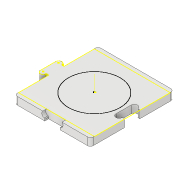
# Autodesk Inventor part: 10_Base_puzzle_sideplate_v3
Saved by Autodesk Inventor 2022 (Build 260153000, 153)
## iProperties
Created: 2017-06-20
Part Number: 10_Base_puzzle_sideplate_v3
Material: Generisch
Document SubType Name: Modeling
Designer: diederichbenedict
Density: 1 g/cm^3
Appearance: Weiß
Mass: 7.87446 g
Surface Area: 71.4468 cm^2
Volume: 7.87446 cm^3
d_part: 50,000 mm
d_o: 40,000 mm
d_i: 40,000 mm
Author: diederichbenedict
Autodesk Inventor part; units mm, degrees
ref_plane "YZ Plane" through (0, 0, 0) normal (1, 0, 0) x (0, 1, 0)
ref_plane "XZ Plane" through (0, 0, 0) normal (0, 1, 0) x (-1, 0, 0)
ref_plane "XY Plane" through (0, 0, 0) normal (0, 0, 1) x (1, 0, 0)
sketch "Skizze1" plane through (0, 0, 0) normal (0, 0, 1) x (1, 0, 0)
  line L0 (-17.4, -0.2) -> (-25.4, -0.2)
  line L1 (-25.4, -0.2) -> (-25.4, -23.2)
  line L2 (-23.4, -25.2) -> (-0.4, -25.2)
  line L3 (-0.4, -25.2) -> (-0.4, -17.2)
  line L4 (-17.4, -0.2) -> (-17.4, -15.2)
  line L5 (-15.4, -17.2) -> (-0.4, -17.2)
  arc A0 (-25.4, -23.2) -> (-23.4, -25.2) centre (-23.4, -23.2) ccw
  circle A1 centre (-20.4, -20.2) radius 2.425
  circle A2 centre (-21.2, -14.7) radius 2.65
  circle A3 centre (-14.9, -21) radius 2.65
  arc A4 (-17.4, -15.2) -> (-15.4, -17.2) centre (-15.4, -15.2) ccw
  circle A5 centre (-20.4, -20.2) radius 2.425
  circle A6 centre (-14.9, -21) radius 2.65
  circle A7 centre (-21.2, -14.7) radius 2.65
  line L6 (-17.4, -0.2) -> (-0.4, -0.2)
  line L7 (-0.4, -0.2) -> (-0.4, -17.2)
  line L8 (-25.4, -23.2) -> (-25.4, -25.2)
  line L9 (-25.4, -25.2) -> (-23.4, -25.2)
  point P0 (-17.4, -17.2)
  dimension "d278" = 25
  dimension "d279" = 25
  dimension "d2" = 8
  dimension "d281" = 8
  dimension "d282" = 2
  dimension "d283" = 4.85
  dimension "d284" = 20
  dimension "d4" = 20
  dimension "d286" = 5.3
  dimension "d_hole" = 5.3
  dimension "d290" = 20.8
  dimension "d" = 20.8
  dimension "d292" = 2
  dimension "d313" = 6.3
  dimension "d314" = 6.3
  dimension "d330" = 0
  dimension "d331" = 0
  dimension "d332" = 0
  constraints: 20 end point, 8 centre point, 5 tangent, 4 point on circle, 4 point on line, 3 horizontal, 2 coincident, 2 parallel, 1 collinear, 1 perpendicular, 1 vertical
  measures "d278" distance of L2.end L8.end
  measures "d279" distance of L8.end L0.end
  measures "d2" distance between parallel lines of L4 L1
  measures "d281" distance between parallel lines of L2 L5
  measures "d282" radius of A0
  measures "d283" diameter of A1
  measures "d284" distance from line of L0 A1.centre
  measures "d4" distance from line of L3 A1.centre
  measures "d286" diameter of A2
  measures "d_hole" diameter of A3
  measures "d290" distance from line of L0 A3.centre
  measures "d" distance from line of L3 A2.centre
  measures "d292" radius of A4
  measures "d313" horizontal distance of A2.centre A3.centre
  measures "d314" horizontal distance of A2.centre A3.centre
  measures "d330" radial gap between concentric circles of A1 A5
  measures "d331" radial gap between concentric circles of A3 A6
  measures "d332" radial gap between concentric circles of A2 A7
extrude "Extrusion1" add sketch "Skizze1" along normal blind 5 contours L4 A4 L5 L3 L2 A0 L1 L0 | L6 L7 L5 A4 L4 | A0 L9 L8 | A1 | A2 | A3
mirror "Mirror6" about plane through (-17.4, -0.2, 0) normal (0, 1, 0) of "Extrusion1"
mirror "Mirror7" about plane through (-0.4, -25.2, 0) normal (1, 0, 0) of "Extrusion1", "Mirror6"
sketch "Sketch26" plane through (0, 0, 5) normal (0, 0, 1) x (1, 0, 0)
  line L0 (24.6, 24.8) -> (-25.4, 24.8) projected
  line L1 (-25.4, -25.2) -> (-25.4, 24.8) projected
  line L2 (-25.4, -25.2) -> (24.6, -25.2) projected
  line L3 (24.6, 24.8) -> (24.6, -25.2) projected
  line L4 (-25.4, -23.2) -> (-25.4, 22.8) projected
  line L5 (-28.9, -7.2) -> (-28.9, -7.2)
  line L6 (-30.9, -5.2) -> (-30.9, 4.8)
  line L7 (-28.9, 6.8) -> (-28.9, 6.8)
  line L8 (-25.4, 6.8) -> (-25.4, -7.2)
  line L9 (-26.9, -5.2) -> (-26.9, 4.8)
  line L10 (-26.4505, 4.8) -> (-25.4, 4.8)
  line L11 (-25.4, 4.8) -> (-25.4, -5.2)
  line L12 (-25.4, -5.2) -> (-26.4505, -5.2)
  line L13 (-26.9, -5.2) -> (-25.4, 4.8) construction
  line L14 (-26.9, 4.8) -> (-25.4, -5.2) construction
  line L15 (-26.9, -5.2) -> (-26.9, -5.2)
  line L16 (-26.9, 4.8) -> (-26.9, 4.8)
  arc A0 (-30.9, -5.2) -> (-28.9, -7.2) centre (-28.9, -5.2) ccw
  arc A1 (-28.9, -7.2) -> (-26.9404, -5.6) centre (-28.9, -5.2) ccw
  arc A2 (-28.9, 6.8) -> (-30.9, 4.8) centre (-28.9, 4.8) ccw
  arc A3 (-26.9404, 5.2) -> (-28.9, 6.8) centre (-28.9, 4.8) ccw
  arc A4 (-26.4505, -5.2) -> (-26.9404, -5.6) centre (-26.4505, -5.7) ccw
  arc A5 (-26.9404, 5.2) -> (-26.4505, 4.8) centre (-26.4505, 5.3) ccw
  point P0 (0, 0)
  point P1 (-26.15, -0.2)
  point P2 (-25.4, -0.2)
  dimension "d293" = 5.5
  dimension "d294" = 14
  dimension "d295" = 18
  dimension "d296" = 10
  dimension "d297" = 1.5
  dimension "d300" = 2
  dimension "d301" = 0.5
  constraints: 24 end point, 14 point on circle, 12 tangent, 6 centre point, 4 equal radius, 4 midpoint, 4 parallel, 3 perpendicular, 3 point on line, 1 horizontal, 1 vertical
  measures "d293" distance between parallel lines of L1 L6
  measures "d294" distance between parallel lines of L5 L7
  measures "d295" distance between parallel lines of L7 L0
  measures "d296" distance of L9.start L9.end
  measures "d297" distance of L9.end L10.end
  measures "d300" radius of A0
  measures "d301" radius of A4
extrude "Extrusion13" add sketch "Sketch26" against normal up to surface (5 mm away) contours L1 L12 A4 A1 A0 L6 A2 A3 A5 L10
sketch "Sketch27" plane through (0, 0, 5) normal (0, 0, 1) x (1, 0, 0)
  line L0 (24.6, 24.8) -> (-25.4, 24.8) projected
  line L1 (-25.4, -25.2) -> (-25.4, -5.2) projected
  line L2 (-26.4505, 4.8) -> (-25.4, 4.8) projected
  arc A0 (-26.9404, 5.2) -> (-26.4505, 4.8) centre (-26.4505, 5.3) ccw projected
  arc A1 (-26.9404, 5.2) -> (-30.9, 4.8) centre (-28.9, 4.8) ccw projected
  line L3 (-30.9, -5.2) -> (-30.9, 4.8) projected
  arc A2 (-30.9, -5.2) -> (-26.9404, -5.6) centre (-28.9, -5.2) ccw projected
  arc A3 (-26.4505, -5.2) -> (-26.9404, -5.6) centre (-26.4505, -5.7) ccw projected
  line L4 (-25.4, -5.2) -> (-26.4505, -5.2) projected
  line L5 (-25.4, 4.8) -> (-25.4, 24.8) projected
  line L6 (-25.4, -25.2) -> (24.6, -25.2) projected
  line L7 (24.6, 24.8) -> (24.6, -25.2) projected
  circle A4 centre (-0.4, -0.2) radius 17
  point P0 (0, 0)
  constraints: 1 centre point
sketch "Sketch28" plane through (0, 0, 5) normal (0, 0, 1) x (1, 0, 0)
  line L0 (24.6, 24.8) -> (-25.4, 24.8) projected
  line L1 (-25.4, -25.2) -> (-25.4, -5.2) projected
  line L2 (-26.4505, 4.8) -> (-25.4, 4.8) projected
  arc A0 (-26.9404, 5.2) -> (-26.4505, 4.8) centre (-26.4505, 5.3) ccw projected
  arc A1 (-26.9404, 5.2) -> (-30.9, 4.8) centre (-28.9, 4.8) ccw projected
  line L3 (-30.9, -5.2) -> (-30.9, 4.8) projected
  arc A2 (-30.9, -5.2) -> (-26.9404, -5.6) centre (-28.9, -5.2) ccw projected
  arc A3 (-26.4505, -5.2) -> (-26.9404, -5.6) centre (-26.4505, -5.7) ccw projected
  line L4 (-25.4, -5.2) -> (-26.4505, -5.2) projected
  line L5 (-25.4, 4.8) -> (-25.4, 24.8) projected
  line L6 (-25.4, -25.2) -> (24.6, -25.2) projected
  line L7 (24.6, 24.8) -> (24.6, -25.2) projected
  line L8 (-25.4, 22.8) -> (-25.4, 4.8) projected
  line L9 (-25.4, -5.2) -> (-25.4, 4.8)
  line L10 (-30.9, -5.2) -> (-30.9, 4.8)
  arc A4 (-30.9, -5.2) -> (-26.9687, -5.7197) centre (-28.9, -5.2) ccw
  arc A5 (-26.9404, 5.2) -> (-30.9, 4.8) centre (-28.9, 4.8) ccw
  line L11 (-25.4, -5.2) -> (-26.2523, -5.2)
  line L12 (-25.4, 4.8) -> (-26.4505, 4.8)
  arc A6 (-26.2523, -5.2) -> (-25.9588, -5.6095) centre (-25.7545, -5.1531) ccw
  arc A7 (-26.9404, 5.2) -> (-26.4505, 4.8) centre (-26.4505, 5.3) ccw
  arc A8 (-26.9404, 5.2) -> (-26.4505, 4.8) centre (-26.4505, 5.3) ccw projected
  line L13 (-26.9404, 5.2) -> (-26.9404, 5.2)
  line L14 (-26.9687, -5.7197) -> (-25.9588, -5.6095)
  line L15 (24.527, -5.0054) -> (24.527, 4.8151)
  line L16 (19.0089, -5.0023) -> (19.0089, 4.8)
  arc A9 (19.0089, -5.0023) -> (22.9683, -5.5256) centre (20.997, -5.2) ccw
  arc A10 (22.9981, 5.203) -> (19.0089, 4.8) centre (21.0238, 4.8) ccw
  line L17 (24.527, -5.0054) -> (23.4703, -5.0054)
  line L18 (24.527, 4.8151) -> (23.4731, 4.8151)
  arc A11 (23.4703, -5.0054) -> (22.9989, -5.4045) centre (23.4777, -5.4921) ccw
  arc A12 (22.9977, 5.2047) -> (23.4731, 4.8151) centre (23.4731, 5.2998) ccw
  line L19 (22.9977, 5.2047) -> (22.9981, 5.203)
  line L20 (22.9683, -5.5256) -> (22.9989, -5.4045)
  line L21 (18.9339, 4.8) -> (18.9339, -4.9986)
  arc A13 (18.9339, -4.9986) -> (23.0417, -5.541) centre (20.997, -5.2) ccw
  line L22 (23.0417, -5.541) -> (23.0722, -5.4203)
  arc A14 (23.4709, -5.0804) -> (23.0722, -5.4203) centre (23.4777, -5.4921) ccw
  line L23 (23.4709, -5.0804) -> (24.602, -5.0804)
  line L24 (24.602, -5.0804) -> (24.602, 4.8901)
  line L25 (24.602, 4.8901) -> (23.4731, 4.8901)
  arc A15 (23.0716, 5.2179) -> (23.4731, 4.8901) centre (23.4731, 5.2998) ccw
  arc A16 (23.0716, 5.2179) -> (18.9339, 4.8) centre (21.0238, 4.8) ccw
  point P0 (0, 0)
  dimension "d307" = 0.075
  dimension "d315" = 0.1946
  dimension "d316" = 0
  dimension "d317" = 0
  dimension "d318" = 0.0901
  constraints: 34 end point, 28 point on circle, 12 centre point, 5 tangent, 4 parallel, 4 vertical, 1 equal radius, 1 point on line, 8 other
  measures "d307" radial gap between concentric circles of A10 A16
  measures "d315" distance between parallel lines of L11 L17
  measures "d316" vertical distance of A9.centre A2.centre
  measures "d317" vertical distance of A10.centre A5.centre
  measures "d318" distance between parallel lines of L2 L25
extrude "Extrusion14" cut sketch "Sketch28" against normal blind 10 contours L7 L23 A14 L22 A13 L21 A16 A15 L25 | L17 A11 L20 A9 L16 A10 A12 L18 L15
sketch "Sketch30" plane through (0, 0, 5) normal (0, 0, 1) x (1, 0, 0)
  line L0 (24.6, 24.8) -> (-25.4, 24.8) construction
  line L1 (-25.4, -25.2) -> (-25.4, -5.2) construction
  line L2 (-26.4505, 4.8) -> (-25.4, 4.8) construction
  arc A0 (-26.9404, 5.2) -> (-26.4505, 4.8) centre (-26.4505, 5.3) ccw construction
  arc A1 (-26.9404, 5.2) -> (-30.9, 4.8) centre (-28.9, 4.8) ccw construction
  line L3 (-30.9, -5.2) -> (-30.9, 4.8) construction
  arc A2 (-30.9, -5.2) -> (-26.9404, -5.6) centre (-28.9, -5.2) ccw construction
  arc A3 (-26.4505, -5.2) -> (-26.9404, -5.6) centre (-26.4505, -5.7) ccw construction
  line L4 (-25.4, -5.2) -> (-26.4505, -5.2) construction
  line L5 (-25.4, 4.8) -> (-25.4, 24.8) construction
  line L6 (-25.4, -25.2) -> (24.6, -25.2) construction
  line L7 (24.6, 24.8) -> (24.6, 4.8901) construction
  line L8 (24.6, -5.0804) -> (23.4709, -5.0804) construction
  arc A4 (23.4709, -5.0804) -> (23.0722, -5.4203) centre (23.4777, -5.4921) ccw construction
  line L9 (23.0722, -5.4203) -> (23.0417, -5.541) construction
  arc A5 (18.9339, -4.9986) -> (23.0417, -5.541) centre (20.997, -5.2) ccw construction
  line L10 (18.9339, -4.9986) -> (18.9339, 4.8) construction
  arc A6 (23.0716, 5.2179) -> (18.9339, 4.8) centre (21.0238, 4.8) ccw construction
  arc A7 (23.0716, 5.2179) -> (23.4731, 4.8901) centre (23.4731, 5.2998) ccw construction
  line L11 (23.4731, 4.8901) -> (24.6, 4.8901) construction
  line L12 (24.6, -5.0804) -> (24.6, -25.2) construction
  line L13 (-28.9, -7.2) -> (-28.9, -7.2)
  line L14 (-30.9, -5.2) -> (-30.9, 4.8)
  line L15 (-28.9, 6.8) -> (-28.9, 6.8)
  line L16 (-26.9, -5.2) -> (-26.9, 4.8)
  line L17 (-26.4505, 4.8) -> (-25.4, 4.8)
  line L18 (-25.4, 4.8) -> (-25.4, -5.2)
  line L19 (-25.4, -5.2) -> (-26.4505, -5.2)
  line L20 (-26.9, -5.2) -> (-25.4, 4.8) construction
  line L21 (-26.9, 4.8) -> (-25.4, -5.2) construction
  line L22 (-26.9, -5.2) -> (-26.9, -5.2)
  line L23 (-26.9, 4.8) -> (-26.9, 4.8)
  arc A8 (-30.9, -5.2) -> (-28.9, -7.2) centre (-28.9, -5.2) ccw
  arc A9 (-28.9, -7.2) -> (-26.9404, -5.6) centre (-28.9, -5.2) ccw
  arc A10 (-28.9, 6.8) -> (-30.9, 4.8) centre (-28.9, 4.8) ccw
  arc A11 (-26.9404, 5.2) -> (-28.9, 6.8) centre (-28.9, 4.8) ccw
  arc A12 (-26.4505, -5.2) -> (-26.9404, -5.6) centre (-26.4505, -5.7) ccw
  arc A13 (-26.9404, 5.2) -> (-26.4505, 4.8) centre (-26.4505, 5.3) ccw
  arc A14 (-28.9, 6.875) -> (-30.975, 4.8) centre (-28.9, 4.8) ccw
  line L24 (-30.975, 4.8) -> (-30.975, -5.2)
  arc A15 (-30.975, -5.2) -> (-29.5327, -7.1762) centre (-28.9, -5.2) ccw
  arc A16 (-29.5327, -7.1762) -> (-26.8669, -5.615) centre (-28.9, -5.2) ccw
  arc A17 (-26.4505, -5.275) -> (-26.8669, -5.615) centre (-26.4505, -5.7) ccw
  line L25 (-26.4505, -5.275) -> (-25.325, -5.275)
  line L26 (-25.325, -5.275) -> (-25.325, 4.875)
  line L27 (-25.325, 4.875) -> (-26.4505, 4.875)
  arc A18 (-26.8669, 5.215) -> (-26.4505, 4.875) centre (-26.4505, 5.3) ccw
  arc A19 (-26.8669, 5.215) -> (-28.9, 6.875) centre (-28.9, 4.8) ccw
  arc A20 (-28.9, 6.8) -> (-30.9, 4.8) centre (-28.9, 4.8) ccw
  line L28 (-30.9, 4.8) -> (-30.9, -5.2)
  arc A21 (-30.9, -5.2) -> (-29.5098, -7.1048) centre (-28.9, -5.2) ccw
  arc A22 (-29.5098, -7.1048) -> (-26.9404, -5.6) centre (-28.9, -5.2) ccw
  arc A23 (-26.4505, -5.2) -> (-26.9404, -5.6) centre (-26.4505, -5.7) ccw
  line L29 (-26.4505, -5.2) -> (-25.4, -5.2)
  line L30 (-25.4, 4.8) -> (-26.4505, 4.8)
  arc A24 (-26.9404, 5.2) -> (-26.4505, 4.8) centre (-26.4505, 5.3) ccw
  arc A25 (-26.9404, 5.2) -> (-28.9, 6.8) centre (-28.9, 4.8) ccw
  line L31 (-25.4, 4.8) -> (-25.4, -5.2)
  line L32 (-26.4505, 4.8) -> (-25.4, 4.8) projected
  line L33 (-25.4, 4.8) -> (-25.4, 4.8)
  line L34 (-25.4, -5.2) -> (-26.4505, -5.2) projected
  line L35 (-25.4, -5.2) -> (-25.4, -5.2)
  arc A26 (22.9977, 5.2047) -> (23.4731, 4.8151) centre (23.4731, 5.2998) ccw
  line L36 (24.527, -5.0054) -> (24.527, 4.8151)
  line L37 (19.0089, -5.0023) -> (19.0089, 4.8)
  line L38 (24.527, -5.0054) -> (23.4703, -5.0054)
  arc A27 (23.4703, -5.0054) -> (22.9989, -5.4045) centre (23.4777, -5.4921) ccw
  line L39 (22.9683, -5.5256) -> (22.9989, -5.4045)
  arc A28 (19.0089, -5.0023) -> (22.9683, -5.5256) centre (20.997, -5.2) ccw
  line L40 (24.527, 4.8151) -> (23.4731, 4.8151)
  line L41 (22.9977, 5.2047) -> (22.9981, 5.203)
  arc A29 (22.9981, 5.203) -> (19.0089, 4.8) centre (21.0238, 4.8) ccw
  line L42 (18.8989, 4.8) -> (18.8989, -4.9969)
  arc A30 (18.8989, -4.9969) -> (23.076, -5.5482) centre (20.997, -5.2) ccw
  line L43 (23.076, -5.5482) -> (23.1065, -5.4276)
  arc A31 (23.4712, -5.1154) -> (23.1065, -5.4276) centre (23.4777, -5.4921) ccw
  line L44 (23.4712, -5.1154) -> (24.637, -5.1154)
  line L45 (24.637, -5.1154) -> (24.637, 4.9251)
  line L46 (24.637, 4.9251) -> (23.4731, 4.9251)
  arc A32 (23.1059, 5.2249) -> (23.4731, 4.9251) centre (23.4731, 5.2998) ccw
  arc A33 (23.1059, 5.2249) -> (18.8989, 4.8) centre (21.0238, 4.8) ccw
  line L47 (24.637, 4.9251) -> (24.637, -5.1154)
  line L48 (24.637, -5.1154) -> (23.4712, -5.1154)
  arc A34 (23.4712, -5.1154) -> (23.1065, -5.4276) centre (23.4777, -5.4921) ccw
  line L49 (23.1065, -5.4276) -> (23.076, -5.5482)
  arc A35 (18.8989, -4.9969) -> (23.076, -5.5482) centre (20.997, -5.2) ccw
  line L50 (18.8989, -4.9969) -> (18.8989, 4.8)
  arc A36 (23.1059, 5.2249) -> (18.8989, 4.8) centre (21.0238, 4.8) ccw
  arc A37 (23.1059, 5.2249) -> (23.4731, 4.9251) centre (23.4731, 5.2998) ccw
  line L51 (23.4731, 4.9251) -> (24.637, 4.9251)
  point P0 (-26.15, -0.2)
  point P1 (-25.4, -0.2)
  dimension "d334" = 14
  dimension "d336" = 10
  dimension "d337" = 1.5
  dimension "d338" = 2
  dimension "d339" = 0.5
  dimension "d340" = 0.075
  dimension "d341" = 0.075
  dimension "d342" = 0.075
  dimension "d343" = 0.075
  dimension "d346" = 0.11
  dimension "d347" = 0
  constraints: 74 end point, 62 point on circle, 30 centre point, 13 tangent, 9 vertical, 8 parallel, 4 equal radius, 3 horizontal, 3 midpoint, 3 perpendicular, 2 collinear, 2 point on line, 38 other
  measures "d334" distance between parallel lines of L13 L15
  measures "d336" distance of L16.start L16.end
  measures "d337" distance of L16.end L17.end
  measures "d338" radius of A8
  measures "d339" radius of A12
  measures "d340" radial gap between concentric circles of A11 A19
  measures "d341" radial gap between concentric circles of A19 A25
  measures "d342" distance between parallel lines of L24 L28
  measures "d343" radial gap between concentric circles of A16 A22
  measures "d346" radial gap between concentric circles of A29 A33
  measures "d347" distance between parallel lines of L45 L47
extrude "Extrusion15" cut sketch "Sketch30" against normal blind 10 contours A26 L40 L36 L38 A27 L39 A28 L37 A29 | A33 A32 L46 L45 L44 A31 L43 A30 L42
sketch "Skizze32" plane through (-23.4, 24.8, 5) normal (0, 1, 0) x (1, 0, 0)
  line L0 (-2, 5) -> (48, 5) projected
  line L1 (48, 0) -> (-2, 0) projected
  circle A0 centre (2, 29.8) radius 2.5 projected
  circle A1 centre (23.4, 51) radius 2.5 projected
  line L2 (27.8804, 6.1291) -> (27.8804, 5) projected
  line L3 (27.8804, 5) -> (46, 5) projected
  arc A2 (46, 5) -> (48, 7) centre (46, 7) ccw projected
  line L4 (48, 24.9099) -> (48, 7) projected
  line L5 (48, 24.9099) -> (46.8731, 24.9099) projected
  arc A3 (46.8731, 24.9099) -> (46.4716, 24.5821) centre (46.8731, 24.5002) ccw projected
  arc A4 (42.3339, 25) -> (46.4716, 24.5821) centre (44.4238, 25) ccw projected
  line L6 (42.3339, 25) -> (42.3339, 34.7986) projected
  arc A5 (46.4417, 35.341) -> (42.3339, 34.7986) centre (44.397, 35) ccw projected
  line L7 (46.4417, 35.341) -> (46.4722, 35.2203) projected
  arc A6 (46.4722, 35.2203) -> (46.8709, 34.8804) centre (46.8777, 35.2921) ccw projected
  line L8 (46.8709, 34.8804) -> (48, 34.8804) projected
  line L9 (48, 53) -> (48, 34.8804) projected
  arc A7 (48, 53) -> (46, 55) centre (46, 53) ccw projected
  line L10 (46, 55) -> (28, 55) projected
  line L11 (28, 55) -> (28, 56.0505) projected
  arc A8 (28.4, 56.5404) -> (28, 56.0505) centre (28.5, 56.0505) ccw projected
  arc A9 (28.4, 56.5404) -> (28, 60.5) centre (28, 58.5) ccw projected
  line L12 (28, 60.5) -> (18, 60.5) projected
  arc A10 (18, 60.5) -> (17.6, 56.5404) centre (18, 58.5) ccw projected
  arc A11 (18, 56.0505) -> (17.6, 56.5404) centre (17.5, 56.0505) ccw projected
  line L13 (18, 56.0505) -> (18, 55) projected
  line L14 (18, 55) -> (0, 55) projected
  arc A12 (0, 55) -> (-2, 53) centre (0, 53) ccw projected
  line L15 (-2, 35) -> (-2, 53) projected
  line L16 (-2, 35) -> (-3.0505, 35) projected
  arc A13 (-3.5404, 35.4) -> (-3.0505, 35) centre (-3.0505, 35.5) ccw projected
  arc A14 (-3.5404, 35.4) -> (-7.5, 35) centre (-5.5, 35) ccw projected
  line L17 (-7.5, 35) -> (-7.5, 25) projected
  arc A15 (-7.5, 25) -> (-3.5404, 24.6) centre (-5.5, 25) ccw projected
  arc A16 (-3.0505, 25) -> (-3.5404, 24.6) centre (-3.0505, 24.5) ccw projected
  line L18 (-3.0505, 25) -> (-2, 25) projected
  line L19 (-2, 7) -> (-2, 25) projected
  arc A17 (-2, 7) -> (0, 5) centre (0, 7) ccw projected
  line L20 (0, 5) -> (17.9099, 5) projected
  line L21 (17.9099, 5) -> (17.9099, 6.1269) projected
  arc A18 (17.9099, 6.1269) -> (17.5821, 6.5284) centre (17.5002, 6.1269) ccw projected
  arc A19 (18, 10.6661) -> (17.5821, 6.5284) centre (18, 8.5762) ccw projected
  line L22 (18, 10.6661) -> (27.7986, 10.6661) projected
  arc A20 (28.341, 6.5583) -> (27.7986, 10.6661) centre (28, 8.603) ccw projected
  line L23 (28.341, 6.5583) -> (28.2203, 6.5278) projected
  arc A21 (28.2203, 6.5278) -> (27.8804, 6.1291) centre (28.2921, 6.1223) ccw projected
  line L24 (8, 13) -> (38, 13) projected
  arc A22 (6, 15) -> (8, 13) centre (8, 15) ccw projected
  line L25 (6, 15) -> (6, 45) projected
  arc A23 (8, 47) -> (6, 45) centre (8, 45) ccw projected
  line L26 (8, 47) -> (38, 47) projected
  arc A24 (40, 45) -> (38, 47) centre (38, 45) ccw projected
  line L27 (40, 45) -> (40, 15) projected
  arc A25 (38, 13) -> (40, 15) centre (38, 15) ccw projected
  circle A26 centre (43, 10) radius 2.425 projected
  circle A27 centre (37.5, 9.2) radius 2.65 projected
  circle A28 centre (43.8, 15.5) radius 2.65 projected
  circle A29 centre (43, 50) radius 2.425 projected
  circle A30 centre (37.5, 50.8) radius 2.65 projected
  circle A31 centre (43.8, 44.5) radius 2.65 projected
  circle A32 centre (3, 10) radius 2.425 projected
  circle A33 centre (8.5, 9.2) radius 2.65 projected
  circle A34 centre (2.2, 15.5) radius 2.65 projected
  circle A35 centre (2.2, 44.5) radius 2.65 projected
  circle A36 centre (8.5, 50.8) radius 2.65 projected
  circle A37 centre (3, 50) radius 2.425 projected
  line L28 (-2, 5) -> (-2, 0) projected
  line L29 (48, 5) -> (48, 0) projected
  line L30 (-2, 0) -> (48, 0)
  line L31 (48, 0) -> (48, 5)
  line L32 (48, 5) -> (-2, 5)
  line L33 (-2, 5) -> (-2, 0)
  line L34 (-2, 5) -> (-2, 0) projected
  line L35 (48, 5) -> (48, 0) projected
  arc A38 (17.9849, 6.1269) -> (17.5971, 6.6019) centre (17.5002, 6.1269) ccw
  line L36 (17.9849, 6.1269) -> (17.9849, 4.925)
  line L37 (17.9849, 4.925) -> (0, 4.925)
  arc A39 (-2.075, 7) -> (0, 4.925) centre (0, 7) ccw
  line L38 (-2.075, 7) -> (-2.075, 24.925)
  line L39 (-2.075, 24.925) -> (-3.0505, 24.925)
  arc A40 (-3.0505, 24.925) -> (-3.4669, 24.585) centre (-3.0505, 24.5) ccw
  arc A41 (-7.575, 25) -> (-3.4669, 24.585) centre (-5.5, 25) ccw
  line L40 (-7.575, 25) -> (-7.575, 35)
  arc A42 (-3.4669, 35.415) -> (-7.575, 35) centre (-5.5, 35) ccw
  arc A43 (-3.4669, 35.415) -> (-3.0505, 35.075) centre (-3.0505, 35.5) ccw
  line L41 (-3.0505, 35.075) -> (-2.075, 35.075)
  line L42 (-2.075, 35.075) -> (-2.075, 53)
  arc A44 (0, 55.075) -> (-2.075, 53) centre (0, 53) ccw
  line L43 (0, 55.075) -> (17.925, 55.075)
  line L44 (17.925, 55.075) -> (17.925, 56.0505)
  arc A45 (17.925, 56.0505) -> (17.585, 56.4669) centre (17.5, 56.0505) ccw
  arc A46 (18, 60.575) -> (17.585, 56.4669) centre (18, 58.5) ccw
  line L45 (18, 60.575) -> (28, 60.575)
  arc A47 (28.415, 56.4669) -> (28, 60.575) centre (28, 58.5) ccw
  arc A48 (28.415, 56.4669) -> (28.075, 56.0505) centre (28.5, 56.0505) ccw
  line L46 (28.075, 56.0505) -> (28.075, 55.075)
  line L47 (28.075, 55.075) -> (46, 55.075)
  arc A49 (48.075, 53) -> (46, 55.075) centre (46, 53) ccw
  line L48 (48.075, 53) -> (48.075, 34.8054)
  line L49 (48.075, 34.8054) -> (46.8703, 34.8054)
  arc A50 (46.3989, 35.2045) -> (46.8703, 34.8054) centre (46.8777, 35.2921) ccw
  line L50 (46.3989, 35.2045) -> (46.3683, 35.3256)
  arc A51 (46.3683, 35.3256) -> (42.4089, 34.8023) centre (44.397, 35) ccw
  line L51 (42.4089, 34.8023) -> (42.4089, 25)
  arc A52 (42.4089, 25) -> (46.3981, 24.5971) centre (44.4238, 25) ccw
  arc A53 (46.8731, 24.9849) -> (46.3981, 24.5971) centre (46.8731, 24.5002) ccw
  line L52 (46.8731, 24.9849) -> (48.075, 24.9849)
  line L53 (48.075, 24.9849) -> (48.075, 7)
  arc A54 (46, 4.925) -> (48.075, 7) centre (46, 7) ccw
  line L54 (46, 4.925) -> (27.8054, 4.925)
  line L55 (27.8054, 4.925) -> (27.8054, 6.1297)
  arc A55 (28.2045, 6.6011) -> (27.8054, 6.1297) centre (28.2921, 6.1223) ccw
  line L56 (28.2045, 6.6011) -> (28.3256, 6.6317)
  arc A56 (28.3256, 6.6317) -> (27.8023, 10.5911) centre (28, 8.603) ccw
  line L57 (27.8023, 10.5911) -> (18, 10.5911)
  arc A57 (18, 10.5911) -> (17.5971, 6.6019) centre (18, 8.5762) ccw
  point P0 (23.4, 5)
  point P1 (27.8054, 5)
  point P2 (17.9849, 5)
  point P3 (-2, 0)
  point P4 (48, 5)
  dimension "d359" = 0.075
  constraints: 52 end point, 40 point on circle, 20 centre point, 2 parallel, 1 horizontal, 1 perpendicular, 41 other
  measures "d359" radial gap between concentric circles of A19 A57
extrude "Extrusion17" add sketch "Skizze32" along normal blind 2.5 contours L0 L36 L37 A39 | A39 L37 L36 L0 L55 L54 A54 L29 L1 L28 | L36 A38 A57 L57 A56 L56 A55 L55 L0 | L0 A54 L54 L55
sketch "Skizze33" plane through (-23.4, -25.2, 0) normal (0, -1, 0) x (1, 0, 0)
  arc A0 (28.4, 1.5404) -> (28, 5.5) centre (28, 3.5) ccw projected
  line L0 (-2, 0) -> (48, 0) projected
  line L1 (-2, 5) -> (48, 5) projected
  line L2 (17.9849, 0) -> (27.8054, 0) projected
  line L3 (46, 0) -> (48, 0) projected
  line L4 (48, 0) -> (48, 5) projected
  line L5 (48, 5) -> (46, 5) projected
  line L6 (46, 0) -> (46, 5) projected
  line L7 (0, 0) -> (-2, 0) projected
  line L8 (0, 0) -> (0, 5) projected
  line L9 (-2, 5) -> (0, 5) projected
  line L10 (-2, 0) -> (-2, 5) projected
  circle A1 centre (2.2, -32.9227) radius 1.5 projected
  line L11 (38, -42) -> (8, -42) projected
  arc A2 (38, -42) -> (40, -40) centre (38, -40) ccw projected
  line L12 (40, -40) -> (40, -10) projected
  arc A3 (40, -10) -> (38, -8) centre (38, -10) ccw projected
  line L13 (23.4, -8) -> (38, -8) projected
  circle A4 centre (23.4, -4) radius 4 projected
  line L14 (8, -8) -> (23.4, -8) projected
  arc A5 (8, -8) -> (6, -10) centre (8, -10) ccw projected
  line L15 (6, -10) -> (6, -25.2) projected
  circle A6 centre (2, -25.2) radius 4 projected
  line L16 (6, -25.2) -> (6, -40) projected
  arc A7 (6, -40) -> (8, -42) centre (8, -40) ccw projected
  circle A8 centre (3, -5) radius 2.425 projected
  circle A9 centre (8.5, -4.2) radius 2.65 projected
  circle A10 centre (2.2, -10.5) radius 2.65 projected
  circle A11 centre (2.2, -39.5) radius 2.65 projected
  circle A12 centre (8.5, -45.8) radius 2.65 projected
  circle A13 centre (3, -45) radius 2.425 projected
  circle A14 centre (43.8, -10.5) radius 2.65 projected
  circle A15 centre (37.5, -4.2) radius 2.65 projected
  circle A16 centre (43, -5) radius 2.425 projected
  circle A17 centre (43.8, -39.5) radius 2.65 projected
  circle A18 centre (37.5, -45.8) radius 2.65 projected
  circle A19 centre (43, -45) radius 2.425 projected
  line L17 (27.8804, -50) -> (27.8804, -48.8709) projected
  arc A20 (28.2203, -48.4722) -> (27.8804, -48.8709) centre (28.2921, -48.8777) ccw projected
  line L18 (28.2203, -48.4722) -> (28.341, -48.4417) projected
  arc A21 (28.341, -48.4417) -> (27.7986, -44.3339) centre (28, -46.397) ccw projected
  line L19 (27.7986, -44.3339) -> (18, -44.3339) projected
  arc A22 (18, -44.3339) -> (17.5821, -48.4716) centre (18, -46.4238) ccw projected
  arc A23 (17.9099, -48.8731) -> (17.5821, -48.4716) centre (17.5002, -48.8731) ccw projected
  line L20 (17.9099, -48.8731) -> (17.9099, -50) projected
  line L21 (17.9099, -50) -> (0, -50) projected
  arc A24 (-2, -48) -> (0, -50) centre (0, -48) ccw projected
  line L22 (-2, -30) -> (-2, -48) projected
  line L23 (-3.0505, -30) -> (-2, -30) projected
  arc A25 (-3.0505, -30) -> (-3.5404, -30.4) centre (-3.0505, -30.5) ccw projected
  arc A26 (-7.5, -30) -> (-3.5404, -30.4) centre (-5.5, -30) ccw projected
  line L24 (-7.5, -20) -> (-7.5, -30) projected
  arc A27 (-3.5404, -19.6) -> (-7.5, -20) centre (-5.5, -20) ccw projected
  arc A28 (-3.5404, -19.6) -> (-3.0505, -20) centre (-3.0505, -19.5) ccw projected
  line L25 (-2, -20) -> (-3.0505, -20) projected
  line L26 (-2, -2) -> (-2, -20) projected
  arc A29 (0, 0) -> (-2, -2) centre (0, -2) ccw projected
  line L27 (0, 0) -> (18, 0) projected
  line L28 (18, 1.0505) -> (18, 0) projected
  arc A30 (18, 1.0505) -> (17.6, 1.5404) centre (17.5, 1.0505) ccw projected
  arc A31 (18, 5.5) -> (17.6, 1.5404) centre (18, 3.5) ccw projected
  line L29 (28, 5.5) -> (18, 5.5) projected
  arc A32 (28.4, 1.5404) -> (28, 5.5) centre (28, 3.5) ccw projected
  arc A33 (28.4, 1.5404) -> (28, 1.0505) centre (28.5, 1.0505) ccw projected
  line L30 (28, 0) -> (28, 1.0505) projected
  line L31 (28, 0) -> (46, 0) projected
  arc A34 (48, -2) -> (46, 0) centre (46, -2) ccw projected
  line L32 (48, -20.1196) -> (48, -2) projected
  line L33 (48, -20.1196) -> (46.8709, -20.1196) projected
  arc A35 (46.4722, -19.7797) -> (46.8709, -20.1196) centre (46.8777, -19.7079) ccw projected
  line L34 (46.4722, -19.7797) -> (46.4417, -19.659) projected
  arc A36 (46.4417, -19.659) -> (42.3339, -20.2014) centre (44.397, -20) ccw projected
  line L35 (42.3339, -20.2014) -> (42.3339, -30) projected
  arc A37 (42.3339, -30) -> (46.4716, -30.4179) centre (44.4238, -30) ccw projected
  arc A38 (46.8731, -30.0901) -> (46.4716, -30.4179) centre (46.8731, -30.4998) ccw projected
  line L36 (46.8731, -30.0901) -> (48, -30.0901) projected
  line L37 (48, -48) -> (48, -30.0901) projected
  arc A39 (46, -50) -> (48, -48) centre (46, -48) ccw projected
  line L38 (46, -50) -> (27.8804, -50) projected
  line L39 (48, 0) -> (48, 5) projected
  line L40 (-2, 0) -> (-2, 5) projected
  line L41 (17.9849, -1.1269) -> (17.9849, 0) projected
  arc A40 (17.5971, -1.6019) -> (17.9849, -1.1269) centre (17.5002, -1.1269) ccw projected
  arc A41 (17.5971, -1.6019) -> (18, -5.5911) centre (18, -3.5762) ccw projected
  line L42 (27.8023, -5.5911) -> (18, -5.5911) projected
  arc A42 (27.8023, -5.5911) -> (28.3256, -1.6317) centre (28, -3.603) ccw projected
  line L43 (28.2045, -1.6011) -> (28.3256, -1.6317) projected
  arc A43 (27.8054, -1.1297) -> (28.2045, -1.6011) centre (28.2921, -1.1223) ccw projected
  line L44 (27.8054, 0) -> (27.8054, -1.1297) projected
  point P0 (23.4, 0)
  point P1 (17.9099, 0)
  point P2 (29.3229, 5)
  point P3 (23.4, 0)
  point P4 (16.6771, 5)
  constraints: 1 horizontal alignment
extrude "Extrusion18" add sketch "Skizze33" along normal blind 2.5 contours A0 L1 L6 L0 L30 A33 | A31 A30 L28 L0 L8 L1 | L1 L4 L0 L6 | L8 L0 L10 L1
fillet "Rundung5" radius 2 4 edges at (24.6, -27.7, 2.5) (-25.4, -27.7, 2.5) (-25.4, 27.3, 2.5) (24.6, 27.3, 2.5)
equation "\"d_i\" = 40"
equation "\"d_o\" = 40"
equation "\"d_part\" = 50"
equation "\"d6\" = 0"
equation "\"d7\" = 0"
equation "\"d8\" = 0"
equation "\"d9\" = 0"
equation "\"d13\" = 0"
equation "\"d14\" = 0"
equation "\"d20\" = 0"
equation "\"d21\" = 0"
equation "\"d22\" = 0"
equation "\"d23\" = 0"
equation "\"d24\" = 0"
equation "\"d25\" = 3"
equation "\"d26\" = 0"
equation "\"d27\" = 0"
equation "\"d28\" = 0"
equation "\"d29\" = 0"
equation "\"d30\" = 0"
equation "\"d31\" = 0"
equation "\"d32\" = 0"
equation "\"d33\" = 0"
equation "\"d34\" = 0"
equation "\"d46\" = 0"
equation "\"d47\" = 0"
equation "\"d48\" = 0"
equation "\"d50\" = 0"
equation "\"d51\" = 0"
equation "\"d52\" = 0"
equation "\"d53\" = 0"
equation "\"d54\" = 0"
equation "\"d55\" = 0"
equation "\"d56\" = 0"
equation "\"d57\" = 0"
equation "\"d58\" = 0"
equation "\"d59\" = 0"
equation "\"magnet_offset\" = 0"
equation "\"screw_offset\" = 0"
equation "\"mal_puzzle_offset\" = 0"
equation "\"fem_puzzle_offset\" = 0"
